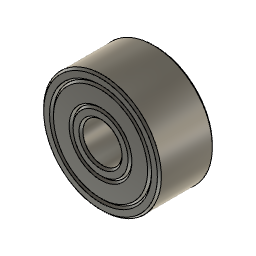
_Lozysko3200.46b5bf71-8898-4d7e-8709-57d1fd050750 (Autodesk Fusion 360 design; units mm, degrees)
Autodesk Fusion 360 part; units mm, degrees
sketch "Sketch1" plane through (0, 0, 0) normal (0, 1, 0) x (1, 0, 0)
  circle A0 centre (0, 0) radius 5
  circle A1 centre (0, 0) radius 7.5
  dimension "d1" = 10
  dimension "d2" = 15
  constraint coincident A0.centre A1.centre
  constraint concentric A0 A1
  measures "d1" diameter of A0
  measures "d2" diameter of A1
extrude "Extrude1" add sketch "Sketch1" along normal blind 14
sketch "Sketch2" plane through (0, 0, 0) normal (0, -1, 0) x (1, 0, 0)
  circle A0 centre (0, 0) radius 5
  circle A1 centre (0, 0) radius 7.5
  circle A2 centre (0, 0) radius 7.5
  circle A3 centre (0, 0) radius 12.5
  dimension "d5" = 25
  constraint concentric A0 A2
  constraint concentric A2 A3
  measures "d5" diameter of A3
chamfer "Chamfer1" distance 0.5 angle 45 2 edges at (-6.9925, 0, 2.7121) (-6.9925, 14, 2.7121)
extrude "Extrude2" add sketch "Sketch2" against normal blind 14 contours A3
chamfer "Chamfer2" distance 0.5 angle 45 4 edges at (-6.9925, 0, 2.7121) (-6.9925, 14, -2.7121) (-11.6541, 14, 4.5202) (-11.6541, 0, -4.5202)
sketch "Sketch3" plane through (0, 0, 0) normal (0, -1, 0) x (1, 0, 0)
  circle A0 centre (0, 0) radius 8
  circle A1 centre (0, 0) radius 12
  circle A2 centre (0, 0) radius 12.5
  circle A3 centre (0, 0) radius 15
  dimension "d10" = 25
  dimension "d11" = 30
  constraint coincident A0.centre A1.centre
  measures "d10" diameter of A2
  measures "d11" diameter of A3
extrude "Extrude3" add sketch "Sketch3" against normal blind 14 contours A3
chamfer "Chamfer3" distance 0.5 angle 45 2 edges at (-11.6541, 0, 4.5202) (-11.6541, 14, -4.5202)
chamfer "Chamfer4" distance 0.5 angle 45 4 edges at (-13.9849, 14, 5.4242) (-13.9849, 0, -5.4242) (-4.6616, 0, -1.8081) (-4.6616, 14, -1.8081)
